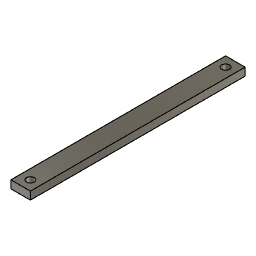
Attacheservo v2 (Autodesk Fusion 360 design; units mm, degrees)
Autodesk Fusion 360 part; units mm, degrees
sketch "Esquisse1" plane through (0, 0, 0) normal (0, 0, 1) x (1, 0, 0)
  line L0 (0, 0) -> (5, 0)
  line L1 (5, 0) -> (5, 55)
  line L2 (5, 55) -> (0, 55)
  line L3 (0, 55) -> (0, 0)
  circle A0 centre (2.5, 52.5) radius 1
  circle A1 centre (2.5, 2.5) radius 1
  dimension "d1" = 55
  dimension "d2" = 5
  dimension "d3" = 2
  dimension "d4" = 2.5
  dimension "d5" = 2.5
  dimension "d6" = 2
  dimension "d7" = 2.5
  dimension "d8" = 2.5
  constraint horizontal L0
  constraint vertical L1
  constraint horizontal L2
  constraint vertical L3
  constraint coincident L0.start L3.end
  measures "d1" distance of L0.end L1.end
  measures "d2" distance of L1.end L2.end
  measures "d3" diameter of A0
  measures "d4" distance of L2 A0.centre
  measures "d5" distance of L3 A0.centre
  measures "d6" diameter of A1
  measures "d7" distance of L1 A1.centre
  measures "d8" distance of L0 A1.centre
extrude "Extrusion1" add sketch "Esquisse1" along normal blind 2
